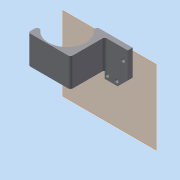
# Autodesk Inventor part: cellSTORM_alviumadapter
Saved by Autodesk Inventor 2019.4 (Build 234330000, 330)
## iProperties
Created: 2020-06-15
Part Number: cellSTORM_alviumadapter
Material: Generic
Document SubType Name: Modeling
Designer: diederichbenedict
Density: 1 g/cm^3
Appearance: Default
Author: diederichbenedict
Autodesk Inventor part; units mm, degrees
ref_plane "YZ Plane" through (0, 0, 0) normal (1, 0, 0) x (0, 1, 0)
ref_plane "XZ Plane" through (0, 0, 0) normal (0, 1, 0) x (-1, 0, 0)
ref_plane "Work Plane1" through (0, 0, 0) normal (0, 0, 1) x (1, 0, 0)
sketch "Sketch1" plane through (0, 0, 0) normal (0, 0, 1) x (1, 0, 0)
  circle A0 centre (2.6061, 6.2821) radius 1.5 construction
  circle A1 centre (22.6061, 6.2821) radius 1.5 construction
  line L0 (-2.6427, 15.6321) -> (-2.6427, -2.7179) construction
  line L1 (-2.6427, -2.7179) -> (30.1061, -2.7179) construction
  line L2 (30.1061, -2.7179) -> (30.1061, -39.6443) construction
  line L3 (30.1061, -39.6443) -> (66.9651, 7.5331) construction
  line L4 (66.9651, 7.5331) -> (66.9651, 15.6321) construction
  line L5 (66.9651, 15.6321) -> (-2.6427, 15.6321) construction
  circle A2 centre (12.3511, 11.6321) radius 1.45 construction
  circle A3 centre (41.9344, -5.4679) radius 1.45 construction
  circle A4 centre (34.1061, -5.4679) radius 1.45 construction
  circle A5 centre (54.6178, 11.6321) radius 1.45 construction
  circle A6 centre (-0.6427, 11.6823) radius 1.45 construction
  circle A7 centre (29.5857, 11.6321) radius 1.45 construction
  circle A8 centre (51.7579, -5.4342) radius 1.45 construction
  circle A9 centre (34.1061, -24.4536) radius 1.45 construction
  circle A10 centre (47.169, 11.6321) radius 1.45 construction
  line L6 (-2.0689, 15.0821) -> (-2.0689, 2.6821) construction
  line L7 (27.2811, 15.0821) -> (27.2811, 2.6821) construction
  line L8 (32.1612, -8.9378) -> (42.8353, -8.9378)
  line L9 (42.8353, -8.9378) -> (51.0915, -0.6816)
  line L10 (51.0915, -0.6816) -> (51.0915, 15.6321)
  line L11 (32.1612, -8.9378) -> (32.1612, 15.6321)
  line L12 (32.1612, 15.6321) -> (51.0915, 15.6321)
  circle A11 centre (34.1061, -5.4679) radius 1.55
  circle A12 centre (41.9344, -5.4679) radius 1.55
  circle A13 centre (47.169, 11.6321) radius 1.55
  line L13 (32.1612, 15.6321) -> (51.0915, 15.6321)
  line L14 (51.0915, 15.6321) -> (51.0915, 20.6321)
  line L15 (51.0915, 20.6321) -> (32.1612, 20.6321)
  line L16 (32.1612, 20.6321) -> (32.1612, 15.6321)
  point P0 (0, 0)
  dimension "d0" = 135
  dimension "d1" = 3.1
  dimension "d2" = 3.1
  dimension "d3" = 3.1
  dimension "d16" = 5
  constraints: 18 end point, 3 centre point, 3 coincident, 2 horizontal, 2 parallel, 2 perpendicular, 1 collinear, 1 midpoint, 1 point on line
  measures "d0" angle of L9 L8
  measures "d1" diameter of A11
  measures "d2" diameter of A12
  measures "d3" diameter of A13
  measures "d16" distance of L14.end L13.end
extrude "Extrusion1" add sketch "Sketch1" along normal blind 4
sketch "Sketch5" plane through (32.1612, 20.6321, 0) normal (0, 1, 0) x (1, 0, 0)
  circle A0 centre (-19.5551, -14.65) radius 15.24 construction
  circle A1 centre (-19.3039, -15.5) radius 15.5 construction
  line L0 (-34.8039, 0) -> (-34.8039, -32) construction
  line L1 (34.8039, 0) -> (-34.8039, 0) construction
  line L2 (0, 0) -> (18.9303, 0) construction
  line L3 (0, 0) -> (0, -4) construction
  line L4 (18.9303, -4) -> (0, -4) construction
  line L5 (18.9303, 0) -> (18.9303, -4) construction
  line L6 (0, 0) -> (18.9303, 0) construction
  line L7 (0, 0) -> (-19.3058, 0) construction
  line L8 (0, 0) -> (-19.3039, 0)
  line L9 (-34.8039, -32) -> (0, -32)
  line L10 (0, -32) -> (0, 0)
  arc A2 (-34.8039, -15.5) -> (-19.3039, 0) centre (-19.3039, -15.5) ccw
  line L11 (-34.8039, -32) -> (-34.8039, -15.5)
  point P0 (-32.1612, 0)
  dimension "d21" = 31
  constraints: 14 end point, 4 point on circle, 4 tangent, 3 centre point, 3 point on line, 2 horizontal, 1 collinear, 1 concentric, 1 perpendicular, 1 vertical, 5 other
  measures "d21" diameter of A1
ref_plane "Work Plane3" through (-2.6427, -2.7179, 0) normal (0, 1, 0) x (0, 0, 1)
extrude "Extrusion5" add sketch "Sketch5" against normal up to surface (23.35 mm away)
fillet "Fillet1" radius 2 5 edges at (-2.6427, 8.9571, 15.5) (12.8573, 8.9571, 0) (32.1612, 8.9571, 32) (-2.6427, 8.9571, 32) (32.1612, 8.9571, 4)
body "Solid1"
